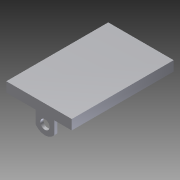
# Autodesk Inventor part: WT11S_terminal
Saved by Autodesk Inventor 2011 SP1 (Build 150282100, 282)
## iProperties
Created: 2013-12-24
Part Number: WT11S_terminal
Catalog Web Link: www.cadenas.de
Description: WT Terminals-WT Terminals
Vendor: NKKSWITCHES
Document SubType Name: Modeling
Designer: PARTuser1
Manufacturer: NKKSWITCHES
Density: 1 g/cm^3
Category: PARTsolutions
Company: NKKSWITCHES
Title: WT11S_terminal
Author: Cadenas PARTsolutions
Comments: WT Terminals
PSOL_IDENT_0: {$CADENAS_DATA\23d-libs\nkkswitches\toggle\wt\parts\wt_terminals.prj},192 {VTYP=3D},{NB=WT11S_termin
PSOL_IDENT_1: al},{LINA=WT11S_terminal},{NN=WT Terminals},{DATE=26.06.2008 06:43:11},{GEOMDATE=26.06.2008 06:43:00
PSOL_IDENT_2: },{VERSION=},{LINEID=10},{LINESUBID=-1},{WBVAR=PLS,CRCTS,TRMNLS}  {NB=WT11S_terminal},{LINA=WT11S_te
PSOL_IDENT_3: rminal},{KT=DUMMY},{PN=WT11S},{SRS=WT},{PLS=1},{CRCTS=1},{TRMNLS=S},{PLSX1=ST}
CNS_NN: WT Terminals
CNS_NT: WT Terminals
CNS_NB: WT11S_terminal
CNS_NBSYN: $PN._terminal
CNS_LINA: WT11S_terminal
CNS_PN: WT11S
CNS_SRS: WT
CNS_PLS: 1 - SPST/SPDT
CNS_CRCTS: 1 - ON/NONE/OFF
CNS_TRMNLS: S - Solder Lug
CNS_PLSX1: ST
SUPPLIER: NKKSWITCHES
ARTICLENO: WT11S_terminal
BOMINFO: WT11S_terminal
CREATOR: CADENAS GmbH
Autodesk Inventor part; units mm, degrees
sketch "Sketch_2" plane through (0, 1.27, 0) normal (0, 1, 0) x (1, 0, 0)
  line L0 (-8.4328, -13.1318) -> (8.4328, -13.1318)
  line L1 (8.4328, -13.1318) -> (8.4328, 13.1318)
  line L2 (8.4328, 13.1318) -> (-8.4328, 13.1318)
  line L3 (-8.4328, 13.1318) -> (-8.4328, -13.1318)
  constraints: 8 end point
extrude "Extrusion1" add sketch "Sketch_2" along normal blind 2.54
sketch "Sketch_1" plane through (0, 0, -11.2014) normal (0, 0, 1) x (1, 0, 0)
  line L0 (-2.4003, 1.27) -> (-2.4003, -3.5306)
  arc A0 (-2.4003, -3.5306) -> (2.4003, -3.5306) centre (0, -1.8973) ccw
  line L1 (2.4003, -3.5306) -> (2.4003, 1.27)
  line L2 (2.4003, 1.27) -> (-2.4003, 1.27)
  circle A1 centre (0, -2.4003) radius 1.1938
  constraints: 6 end point, 2 centre point, 2 point on circle
extrude "Extrusion2" add sketch "Sketch_1" along normal mid plane 0.7874
sketch "Sketch_3" plane through (0, 0, 11.2014) normal (0, 0, 1) x (1, 0, 0)
  line L0 (-2.4003, 1.27) -> (-2.4003, -3.5306)
  arc A0 (-2.4003, -3.5306) -> (2.4003, -3.5306) centre (0, -1.8973) ccw
  line L1 (2.4003, -3.5306) -> (2.4003, 1.27)
  line L2 (2.4003, 1.27) -> (-2.4003, 1.27)
  circle A1 centre (0, -2.4003) radius 1.1938
  constraints: 6 end point, 2 centre point, 2 point on circle
extrude "Extrusion3" add sketch "Sketch_3" along normal mid plane 0.7874
ref_plane "body_to_terminal_XY" through (0, 0, 0) normal (0, -1, 0) x (1, 0, 0)
ref_plane "body_to_terminal_YZ" through (0, 0, 0) normal (1, 0, 0) x (0, 0, 1)
ref_plane "body_to_terminal_ZX" through (0, 0, 0) normal (0, 0, 1) x (0, -1, 0)
ref_plane "wire_1_XY" through (-3.048, 0, 7.62) normal (0, 1, 0) x (1, 0, 0)
ref_plane "wire_1_YZ" through (-3.048, 0, 7.62) normal (1, 0, 0) x (0, 0, -1)
ref_plane "wire_1_ZX" through (-3.048, 0, 7.62) normal (0, 0, -1) x (0, 1, 0)
ref_plane "wire_2_XY" through (3.048, 0, 7.62) normal (0, 1, 0) x (1, 0, 0)
ref_plane "wire_2_YZ" through (3.048, 0, 7.62) normal (1, 0, 0) x (0, 0, -1)
ref_plane "wire_2_ZX" through (3.048, 0, 7.62) normal (0, 0, -1) x (0, 1, 0)
ref_plane "wire_3_XY" through (-3.048, 0, 0) normal (0, 1, 0) x (1, 0, 0)
ref_plane "wire_3_YZ" through (-3.048, 0, 0) normal (1, 0, 0) x (0, 0, -1)
ref_plane "wire_3_ZX" through (-3.048, 0, 0) normal (0, 0, -1) x (0, 1, 0)
ref_plane "wire_4_XY" through (3.048, 0, 0) normal (0, 1, 0) x (1, 0, 0)
ref_plane "wire_4_YZ" through (3.048, 0, 0) normal (1, 0, 0) x (0, 0, -1)
ref_plane "wire_4_ZX" through (3.048, 0, 0) normal (0, 0, -1) x (0, 1, 0)
ref_plane "wire_5_XY" through (-3.048, 0, -7.62) normal (0, 1, 0) x (1, 0, 0)
ref_plane "wire_5_YZ" through (-3.048, 0, -7.62) normal (1, 0, 0) x (0, 0, -1)
ref_plane "wire_5_ZX" through (-3.048, 0, -7.62) normal (0, 0, -1) x (0, 1, 0)
ref_plane "wire_6_XY" through (3.048, 0, -7.62) normal (0, 1, 0) x (1, 0, 0)
ref_plane "wire_6_YZ" through (3.048, 0, -7.62) normal (1, 0, 0) x (0, 0, -1)
ref_plane "wire_6_ZX" through (3.048, 0, -7.62) normal (0, 0, -1) x (0, 1, 0)
body "Solid1"
